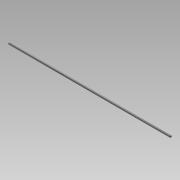
# Autodesk Inventor part: DD_KVD_002_08
Saved by Autodesk Inventor 2017.3 (Build 213256000, 256)
## iProperties
Created: 2023-12-12
Part Number: DD_KVD_002_08
Material: Nerezová ocel
Document SubType Name: Modeling
Designer: Darena
Manufacturer: Standard
Standards Organization: Custom
Density: 8 g/cm^3
Appearance: Pololeštěná
Author: Darena
Autodesk Inventor part; units mm, degrees
ref_plane "YZ Plane" through (0, 0, 0) normal (1, 0, 0) x (0, 1, 0)
ref_plane "XZ Plane" through (0, 0, 0) normal (0, 1, 0) x (-1, 0, 0)
ref_plane "XY Plane" through (0, 0, 0) normal (0, 0, 1) x (1, 0, 0)
sketch "Náčrt3" plane through (0, 0, 0) normal (1, 0, 0) x (0, 1, 0)
  circle A0 centre (0, 0) radius 6.5
  dimension "d16" = 13
  constraints: 1 centre point, 1 coincident
  measures "d16" diameter of A0
extrude "Vysunutí1" add sketch "Náčrt3" along normal mid plane 1055
chamfer "Zkosení2" distance 1 angle 45 2 edges at (527.5, -6.5, 0) (-527.5, -6.5, 0)
